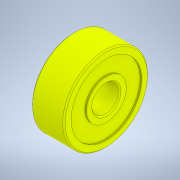
# Autodesk Inventor part: idl-bearing
Saved by Autodesk Inventor 2020 (Build 240168000, 168)
## iProperties
Created: 2020-10-21
Part Number: idl-bearing
Material: Generic
Document SubType Name: Modeling
Designer: alnwlsn
Density: 1 g/cm^3
Appearance: Default
Author: alnwlsn
Autodesk Inventor part; units mm, degrees
ref_plane "YZ Plane" through (0, 0, 0) normal (1, 0, 0) x (0, 1, 0)
ref_plane "XZ Plane" through (0, 0, 0) normal (0, 1, 0) x (-1, 0, 0)
ref_plane "XY Plane" through (0, 0, 0) normal (0, 0, 1) x (1, 0, 0)
sketch "Sketch2" plane through (0, 0, 0) normal (0, 1, 0) x (-1, 0, 0)
  line L0 (0, 0) -> (10.4128, 0) construction
  line L1 (0, -2.05) -> (5, -2.05)
  line L2 (5, -2.05) -> (5, -3.065)
  line L3 (5, -3.065) -> (4.8, -3.065)
  line L4 (4.8, -3.065) -> (4.8, -5.4)
  line L5 (4.8, -5.4) -> (5, -5.4)
  line L6 (5, -5.4) -> (5, -6.5)
  line L7 (5, -6.5) -> (0, -6.5)
  line L8 (0, -6.5) -> (0, -5.4)
  line L9 (0, -5.4) -> (0.2, -5.4)
  line L10 (0.2, -5.4) -> (0.2, -3.065)
  line L11 (0.2, -3.065) -> (0, -3.065)
  line L12 (0, -2.05) -> (0, -3.065)
  dimension "d0" = 5
  dimension "d1" = 2.05
  dimension "d2" = 3.065
  dimension "d3" = 5.4
  dimension "d4" = 6.5
  dimension "d5" = 0.2
  constraints: 26 end point, 9 perpendicular, 6 point on line, 2 collinear, 2 horizontal
  measures "d0" distance of L6.end L7.end
  measures "d1" distance between parallel lines of L0 L1
  measures "d2" distance between parallel lines of L0 L3
  measures "d3" distance between parallel lines of L0 L5
  measures "d4" distance between parallel lines of L0 L7
  measures "d5" distance between parallel lines of L6 L4
revolve "Revolution1" add sketch "Sketch2" angle 360 about axis through (0, 0, 0) along (-1, 0, 0)
chamfer "Chamfer1" distance 0.2 angle 45 4 edges at (0, 0, 6.5) (-5, 0, 6.5) (0, 0, 2.05) (-5, 0, 2.05)
body "Solid1"
